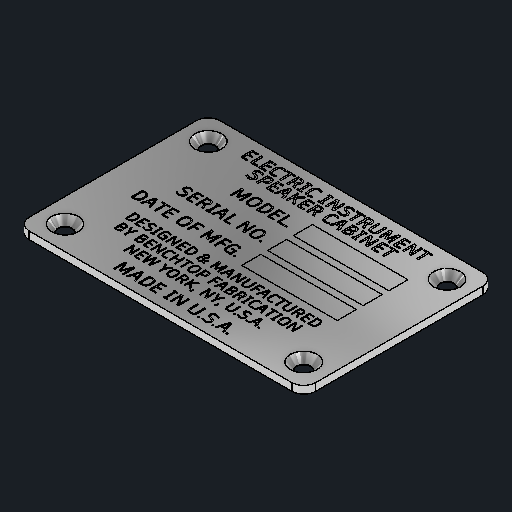
# Autodesk Inventor part: Jack Plate
Saved by Autodesk Inventor 2026.2 (Build 302298000, 298)
## iProperties
Created: 2026-06-24
Part Number: Jack Plate
Material: Aluminum 6061
Document SubType Name: Sheet Metal
Designer: JoshuaEah
Density: 2.7 g/cm^3
Sheet Metal Rule: Default_mm
Appearance: Chrome - Polished
Author: JoshuaEah
Autodesk Inventor part; units mm, degrees
ref_plane "YZ Plane" through (0, 0, 0) normal (1, 0, 0) x (0, 1, 0)
ref_plane "XZ Plane" through (0, 0, 0) normal (0, 1, 0) x (-1, 0, 0)
ref_plane "XY Plane" through (0, 0, 0) normal (0, 0, 1) x (1, 0, 0)
sketch "Sketch1" plane through (0, 0, 0) normal (0, 1, 0) x (-1, 0, 0)
  line L0 (0, 0) -> (-76.2, 0)
  line L1 (-76.2, 0) -> (-76.2, -50.8)
  line L2 (-76.2, -50.8) -> (0, -50.8)
  line L3 (0, -50.8) -> (0, 0)
  line L4 (0, -25.4) -> (-76.2, -25.4)
  line L5 (-38.1, -50.8) -> (-38.1, 0)
  line L6 (-6.35, -44.45) -> (-69.85, -44.45) construction
  line L7 (-69.85, -44.45) -> (-69.85, -6.35) construction
  line L8 (-69.85, -6.35) -> (-6.35, -6.35) construction
  line L9 (-6.35, -6.35) -> (-6.35, -44.45) construction
  line L10 (-6.35, -44.45) -> (-69.85, -6.35) construction
  line L11 (-69.85, -44.45) -> (-6.35, -6.35) construction
  point P0 (-38.1, -25.4)
  dimension "d0" = 76.2
  dimension "d1" = 50.8
  dimension "d2" = 63.5
  dimension "d3" = 38.1
  constraints: 24 end point, 6 midpoint, 4 coincident, 4 parallel, 2 horizontal, 2 perpendicular, 2 point on line
  measures "d0" distance of L2.end L1.end
  measures "d1" distance of L1.end L0.end
  measures "d2" distance of L7.end L8.end
  measures "d3" distance of L6.end L7.end
extrude "Plate1" add sketch "Sketch1" against normal blind 2
hole "Mounting Hole" at (6.35, 0, -44.45) direction (0, -1, 0) diameter 3.81 end through all countersink diameter 7.0866 countersink angle 82 clearance for "Flat Head Machine Screw (82)" size "#6" standard "Ansi Unified Screw Threads"
pattern_sketch "Mounting Holes" of "Mounting Hole" from (6.35, 0, -44.45) copies at (69.85, 0, -44.45) at (69.85, 0, -6.35) at (6.35, 0, -6.35)
fillet "Corner Round1" radius 3.175 4 edges at (0, -1, -50.8) (76.2, -1, -50.8) (76.2, -1, 0) (0, -1, 0)
sketch "Sketch2" plane through (0, 0, 0) normal (0, 1, 0) x (1, 0, 0)
  line L0 (5.9151, 38.1317) -> (36.83, 38.1317) construction
  line L1 (36.83, 38.1317) -> (36.83, 35.0837) construction
  line L2 (36.83, 35.0837) -> (5.9151, 35.0837) construction
  line L3 (5.9151, 35.0837) -> (5.9151, 38.1317) construction
  line L4 (5.9151, 31.2737) -> (36.83, 31.2737) construction
  line L5 (36.83, 31.2737) -> (36.83, 28.2258) construction
  line L6 (36.83, 28.2258) -> (5.9151, 28.2257) construction
  line L7 (5.9151, 28.2257) -> (5.9151, 31.2737) construction
  line L8 (11.7398, 18.288) -> (64.4602, 18.288) construction
  line L9 (64.4602, 18.288) -> (64.4602, 8.128) construction
  line L10 (64.4602, 8.128) -> (11.7398, 8.128) construction
  line L11 (11.7398, 8.128) -> (11.7398, 18.288) construction
  line L12 (21.6232, 5.588) -> (54.5768, 5.588) construction
  line L13 (54.5768, 5.588) -> (54.5768, 2.54) construction
  line L14 (54.5768, 2.54) -> (21.6232, 2.54) construction
  line L15 (21.6232, 2.54) -> (21.6232, 5.588) construction
  line L16 (5.9151, 24.4157) -> (36.83, 24.4157) construction
  line L17 (36.83, 24.4157) -> (36.83, 21.3677) construction
  line L18 (36.83, 21.3677) -> (5.9151, 21.3677) construction
  line L19 (5.9151, 21.3677) -> (5.9151, 24.4157) construction
  circle A0 centre (6.35, 6.35) radius 3.5433 construction
  circle A1 centre (69.85, 6.35) radius 3.5433 construction
  circle A2 centre (69.85, 44.45) radius 3.5433 construction
  circle A3 centre (6.35, 44.45) radius 3.5433 construction
  arc A4 (0, 3.175) -> (3.175, 0) centre (3.175, 3.175) ccw construction
  line L20 (3.175, 0) -> (73.025, 0) construction
  arc A5 (73.025, 0) -> (76.2, 3.175) centre (73.025, 3.175) ccw construction
  line L21 (76.2, 3.175) -> (76.2, 47.625) construction
  arc A6 (76.2, 47.625) -> (73.025, 50.8) centre (73.025, 47.625) ccw construction
  line L22 (73.025, 50.8) -> (3.175, 50.8) construction
  arc A7 (3.175, 50.8) -> (0, 47.625) centre (3.175, 47.625) ccw construction
  line L23 (0, 47.625) -> (0, 3.175) construction
  circle A8 centre (6.35, 44.45) radius 6.35 construction
  line L24 (73.025, 50.8) -> (3.175, 50.8) projected
  line L25 (38.1, 50.8) -> (38.1, 0) construction
  line L26 (0, 25.4) -> (76.2, 25.4) construction
  circle A9 centre (69.85, 44.45) radius 6.35 construction
  circle A10 centre (6.35, 6.35) radius 6.35 construction
  circle A11 centre (69.85, 6.35) radius 6.35 construction
  line L27 (39.37, 39.1478) -> (64.77, 39.1478)
  line L28 (64.77, 39.1478) -> (64.77, 34.0678)
  line L29 (64.77, 34.0678) -> (39.37, 34.0677)
  line L30 (39.37, 34.0677) -> (39.37, 39.1478)
  line L31 (39.37, 32.2897) -> (64.77, 32.2898)
  line L32 (64.77, 32.2898) -> (64.77, 27.2097)
  line L33 (64.77, 27.2097) -> (39.37, 27.2097)
  line L34 (39.37, 27.2097) -> (39.37, 32.2897)
  line L35 (39.37, 25.4317) -> (64.77, 25.4318)
  line L36 (64.77, 25.4318) -> (64.77, 20.3517)
  line L37 (64.77, 20.3517) -> (39.37, 20.3517)
  line L38 (39.37, 20.3517) -> (39.37, 25.4317)
  line L39 (13.2579, 48.26) -> (62.9421, 48.26) construction
  line L40 (62.9421, 48.26) -> (62.9421, 41.2115) construction
  line L41 (62.9421, 41.2115) -> (13.2579, 41.2115) construction
  line L42 (13.2579, 41.2115) -> (13.2579, 48.26) construction
  point P0 (38.1, 18.288)
  point P1 (38.1, 25.4)
  point P2 (38.1, 5.588)
  point P3 (38.1, 25.4)
  point P4 (39.37, 22.8917)
  point P5 (36.83, 22.8917)
  point P6 (39.37, 29.7497)
  point P7 (36.83, 29.7497)
  point P8 (39.37, 36.6077)
  point P9 (36.83, 36.6077)
  point P10 (38.1, 41.2115)
  dimension "d24" = 2.54
  dimension "d25" = 3.048
  dimension "d26" = 10.16
  dimension "d27" = 2.54
  dimension "d28" = 3.048
  dimension "d29" = 3.048
  dimension "d30" = 3.048
  dimension "d31" = 3.81
  dimension "d32" = 3.81
  dimension "d33" = 2.54
  dimension "d34" = 3.0798
  dimension "d35" = 2.54
  dimension "d36" = 25.4
  dimension "d37" = 5.08
  dimension "d38" = 7.0485
  dimension "d39" = 2.54
  dimension "d40" = 3.0798
  constraints: 28 end point, 15 midpoint, 8 collinear, 7 parallel, 4 centre point, 3 horizontal, 3 horizontal alignment, 3 perpendicular, 3 symmetric about line, 3 vertical alignment, 2 point on line, 1 tangent, 15 other
  measures "d24" distance between parallel lines of L20 L14
  measures "d25" distance of L12.end L13.end
  measures "d26" distance of L8.end L9.end
  measures "d27" distance between parallel lines of L12 L10
  measures "d28" distance of L6.end L4.start
  measures "d29" distance of L18.end L16.start
  measures "d30" distance of L2.end L0.start
  measures "d31" distance between parallel lines of L2 L4
  measures "d32" distance between parallel lines of L16 L6
  measures "d33" distance between parallel lines of L30 L1
  measures "d34" distance between parallel lines of L18 L8
  measures "d35" diameter of L1 L25
  measures "d36" distance of L27.start L27.end
  measures "d37" distance of L27.end L28.end
  measures "d38" distance of L39.end L40.end
  measures "d39" distance between parallel lines of L24 L39
  measures "d40" distance between parallel lines of L41 L0
mark "Mark1"
equation "\"d11\" = Thickness"
equation "\"d5\" = Thickness"
equation "\"largeTextHeight\" = 3.048"
equation "\"smallTextHeight\" = 2.54"
equation "\"Thickness\" = 2"
body "Solid1"
